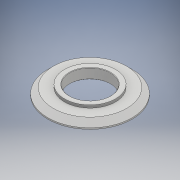
# Autodesk Inventor part: KMB602PT-機械油封墊片
Saved by Autodesk Inventor 2018 (Build 220112000, 112)
## iProperties
Created: 2024-12-13
Part Number: KMB602PT-機械油封墊片
Material: 一般
Document SubType Name: Modeling
Designer: User
Density: 1 g/cm^3
Appearance: 預設
Author: User
Autodesk Inventor part; units mm, degrees
ref_plane "YZ Plane" through (0, 0, 0) normal (1, 0, 0) x (0, 1, 0)
ref_plane "XZ Plane" through (0, 0, 0) normal (0, 1, 0) x (-1, 0, 0)
ref_plane "XY Plane" through (0, 0, 0) normal (0, 0, 1) x (1, 0, 0)
sketch "草圖1" plane through (0, 0, 0) normal (0, 0, 1) x (1, 0, 0)
  circle A0 centre (0, 0) radius 31.05
  dimension "d0" = 62.1
  constraints: 1 centre point, 1 coincident
  measures "d0" diameter of A0
extrude "擠出1" add sketch "草圖1" along normal blind 5
sketch "草圖2" plane through (0, 0, 5) normal (0, 0, 1) x (1, 0, 0)
  circle A0 centre (0, 0) radius 18.85
  dimension "d3" = 37.7
  constraints: 1 centre point, 1 coincident
  measures "d3" diameter of A0
extrude "擠出2" add sketch "草圖2" along normal blind 2
sketch "草圖3" plane through (0, 0, 0) normal (0, 0, -1) x (-1, 0, 0)
  circle A0 centre (0, 0) radius 20
  dimension "d6" = 40
  constraints: 1 centre point, 1 coincident
  measures "d6" diameter of A0
extrude "擠出3" add sketch "草圖3" along normal blind 0.5
sketch "草圖4" plane through (0, 0, 7) normal (0, 0, 1) x (1, 0, 0)
  circle A0 centre (0, 0) radius 15
  dimension "d9" = 30
  constraints: 1 centre point, 1 coincident
  measures "d9" diameter of A0
extrude "擠出4" cut sketch "草圖4" against normal blind 7.5
chamfer "倒角1" distance 4 angle 45 1 edges at (-31.05, 0, 5)
chamfer "倒角2" distance 0.3 angle 45 2 edges at (-15, 0, 7) (-15, 0, -0.5)
